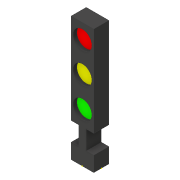
# Autodesk Inventor part: trafficlight
Saved by Autodesk Inventor 2018 (Build 220112000, 112)
## iProperties
Created: 2017-08-24
Part Number: trafficlight
Material: Generic
Document SubType Name: Modeling
Designer: Platform
Density: 1 g/cm^3
Appearance: Default
Author: Platform
Autodesk Inventor part; units mm, degrees
ref_plane "YZ Plane" through (0, 0, 0) normal (1, 0, 0) x (0, 1, 0)
ref_plane "XZ Plane" through (0, 0, 0) normal (0, 1, 0) x (-1, 0, 0)
ref_plane "XY Plane" through (0, 0, 0) normal (0, 0, 1) x (1, 0, 0)
sketch "Sketch1" plane through (0, 0, 0) normal (0, 0, 1) x (1, 0, 0)
  point P0 (0, 0)
sketch "Sketch2" plane through (0, 0, 0) normal (0, 0, 1) x (1, 0, 0)
  line L0 (-15, 20) -> (15, 20)
  line L1 (15, 20) -> (15, 0)
  line L2 (15, 0) -> (-15, 0)
  line L3 (-15, 0) -> (-15, 20)
  point P0 (0, 0)
  dimension "d0" = 30
  dimension "d1" = 20
  dimension "d2" = 20
  dimension "d3" = 15
  constraints: 8 end point, 2 parallel, 1 horizontal, 1 perpendicular
  measures "d0" distance of L1.end L2.end
  measures "d1" distance of L0.end L1.end
  measures "d2" vertical distance of point (0, 0) L0.start
  measures "d3" distance of L2.end point (0, 0)
extrude "Extrusion1" add sketch "Sketch2" along normal mid plane 20
sketch "Sketch3" plane through (0, 0, 10) normal (0, 0, 1) x (1, 0, 0)
  line L0 (-5, 45) -> (5, 45)
  line L1 (5, 45) -> (5, 20)
  line L2 (5, 20) -> (-5, 20)
  line L3 (-5, 20) -> (-5, 45)
  line L4 (15, 20) -> (-15, 20) projected
  point P0 (0, 0)
  dimension "d6" = 10
  dimension "d7" = 25
  dimension "d8" = 0
  dimension "d9" = 5
  constraints: 8 end point, 2 parallel, 1 horizontal, 1 perpendicular
  measures "d6" distance of L1.end L2.end
  measures "d7" distance of L0.end L1.end
  measures "d8" distance between parallel lines of L4 L2
  measures "d9" horizontal distance of point (0, 0) L2.end
extrude "Extrusion2" add sketch "Sketch3" against normal blind 20
sketch "Sketch4" plane through (0, 0, 10) normal (0, 0, 1) x (1, 0, 0)
  line L0 (-15, 165) -> (15, 165)
  line L1 (15, 165) -> (15, 45)
  line L2 (15, 45) -> (-15, 45)
  line L3 (-15, 45) -> (-15, 165)
  line L4 (-5, 45) -> (5, 45) projected
  point P0 (0, 0)
  dimension "d12" = 30
  dimension "d13" = 120
  dimension "d14" = 0
  dimension "d15" = 15
  constraints: 8 end point, 2 parallel, 1 horizontal, 1 perpendicular
  measures "d12" distance of L1.end L2.end
  measures "d13" distance of L0.end L1.end
  measures "d14" distance between parallel lines of L4 L2
  measures "d15" horizontal distance of L2.end point (0, 0)
extrude "Extrusion3" add sketch "Sketch4" against normal blind 20
sketch "Sketch5" plane through (0, 0, 10) normal (0, 0, 1) x (1, 0, 0)
  point P0 (0, 0)
sketch "Sketch6" plane through (0, 0, 10) normal (0, 0, 1) x (1, 0, 0)
  line L0 (0, 45) -> (0, 165)
  line L1 (-15, 165) -> (15, 165) projected
  line L2 (0, 165) -> (0, 125)
  line L3 (0, 125) -> (0, 85)
  line L4 (0, 85) -> (0, 45)
  line L5 (0, 165) -> (0, 145)
  line L6 (0, 125) -> (0, 105)
  line L7 (0, 85) -> (0, 65)
  line L8 (0, 165) -> (0, 145)
  circle A0 centre (0, 145) radius 12.5
  point P0 (0, 0)
  dimension "d18" = 40
  dimension "d19" = 40
  dimension "d20" = 20
  dimension "d21" = 20
  dimension "d22" = 20
  dimension "d23" = 25
  constraints: 16 end point, 4 midpoint, 2 collinear, 2 point on line, 1 centre point, 1 coincident
  measures "d18" distance of L0.end L2.end
  measures "d19" distance of L2.end L3.end
  measures "d20" distance of L2.end L6.end
  measures "d21" distance of L3.end L7.end
  measures "d22" distance of L0.end L5.end
  measures "d23" diameter of A0
extrude "Extrusion4" cut sketch "Sketch6" against normal blind 5
sketch "Sketch7" plane through (0, 0, 10) normal (0, 0, 1) x (1, 0, 0)
  line L0 (-15, 165) -> (15, 165) projected
  line L1 (0, 165) -> (0, 105)
  circle A0 centre (0, 105) radius 12.5
  point P0 (0, 0)
  dimension "d26" = 60
  dimension "d27" = 25
  constraints: 2 end point, 1 centre point, 1 coincident, 1 midpoint, 1 vertical
  measures "d26" distance of L1.start L1.end
  measures "d27" diameter of A0
extrude "Extrusion5" cut sketch "Sketch7" against normal blind 5
sketch "Sketch8" plane through (0, 0, 10) normal (0, 0, 1) x (1, 0, 0)
  line L0 (0, 45) -> (0, 65)
  circle A0 centre (0, 65) radius 12.5
  point P0 (0, 0)
  dimension "d30" = 20
  dimension "d31" = 25
  constraints: 2 end point, 1 centre point, 1 coincident, 1 vertical
  measures "d30" distance of L0.start L0.end
  measures "d31" diameter of A0
extrude "Extrusion6" cut sketch "Sketch8" against normal blind 5
sketch "Sketch9" plane through (15, 45, 10) normal (1, 0, 0) x (0, 0, -1)
  point P0 (10, -45)
sketch "Sketch10" plane through (0, 0, 10) normal (0, 0, 1) x (1, 0, 0)
  point P0 (0, 0)
body "Solid1"
